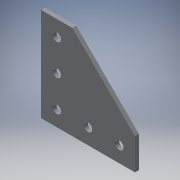
# Autodesk Inventor part: gusset plate
Saved by Autodesk Inventor 2016 (Build 200138000, 138)
## iProperties
Created: 2016-02-03
Part Number: gusset plate
Material: Aluminum 6061
Document SubType Name: Modeling
Designer: gus
Mass: 37.182 g
Surface Area: 98.8447 cm^2
Volume: 13.7711 cm^3
Density: 2.7 g/cm^3
Appearance: Aluminum - Flat
Author: gus
Autodesk Inventor part; units mm, degrees
ref_plane "YZ Plane" through (0, 0, 0) normal (1, 0, 0) x (0, 1, 0)
ref_plane "XZ Plane" through (0, 0, 0) normal (0, 1, 0) x (-1, 0, 0)
ref_plane "XY Plane" through (0, 0, 0) normal (0, 0, 1) x (1, 0, 0)
sketch "Sketch1" plane through (0, 0, 0) normal (0, 0, 1) x (1, 0, 0)
  line L0 (0, 0) -> (76.2, 0)
  line L1 (76.2, 0) -> (76.2, 25.4)
  line L2 (76.2, 25.4) -> (25.4, 76.2)
  line L3 (25.4, 76.2) -> (0, 76.2)
  line L4 (0, 76.2) -> (0, 0)
  circle A0 centre (63.5, 12.7) radius 3.3734
  circle A1 centre (38.1, 12.7) radius 3.3734
  circle A2 centre (12.7, 12.7) radius 3.3734
  circle A3 centre (12.7, 38.1) radius 3.3734
  circle A4 centre (12.7, 63.5) radius 3.3734
  line L5 (0, 12.7) -> (76.2, 12.7) construction
  line L6 (12.7, 0) -> (12.7, 76.2) construction
  dimension "d0" = 76.2
  dimension "d1" = 25.4
  dimension "d2" = 25.4
  dimension "d3" = 76.2
  dimension "d6" = 6.7469
  dimension "d10" = 38.1
  dimension "d11" = 63.5
  dimension "d12" = 38.1
  dimension "d15" = 12.7
  dimension "d16" = 12.7
  dimension "d17" = 63.5
  constraints: 14 end point, 6 point on line, 5 centre point, 4 equal radius, 4 midpoint, 2 perpendicular, 1 horizontal, 1 parallel
  measures "d0" distance of L0.start L0.end
  measures "d1" distance of L0.end L1.end
  measures "d2" distance of L2.end L3.end
  measures "d3" distance of L3.end L0.start
  measures "d6" diameter of A2
  measures "d10" distance from line of L0 A3.centre
  measures "d11" distance from line of L0 A4.centre
  measures "d12" distance from line of A1.centre L4
  measures "d15" distance of L0.start L5.start
  measures "d16" distance of L0.start L6.start
  measures "d17" distance from line of L4 A0.centre
extrude "Extrusion1" add sketch "Sketch1" along normal blind 3.175
body "Solid1"
